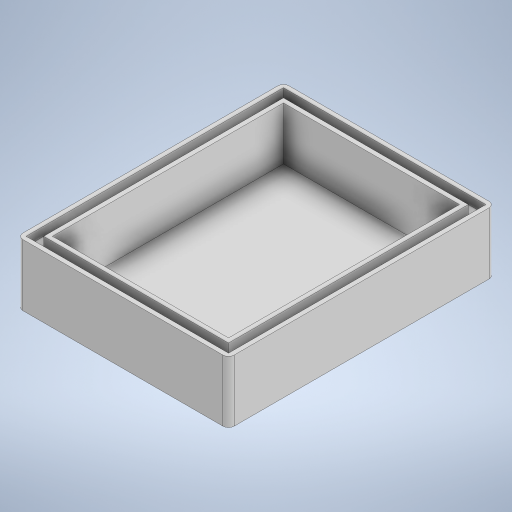
# Autodesk Inventor part: Light Sensor Box V1
Saved by Autodesk Inventor 2024.2 (Build 282272000, 272)
## iProperties
Created: 2024-07-12
Part Number: Light Sensor Box V1
Material: Generic
Document SubType Name: Modeling
Designer: balmo
Density: 1 g/cm^3
Appearance: Default
Author: balmo
## iProperties of the stored document Light Sensor Box V1_3DPrint.ipt
Created: 2024-07-12
Part Number: Light Sensor Box V1_3DPrint
Material: Generic
Document SubType Name: Modeling
Designer: balmo
Density: 1 g/cm^3
Appearance: Default
Author: balmo
Autodesk Inventor part; units mm, degrees
ref_plane "YZ Plane" through (0, 0, 0) normal (1, 0, 0) x (0, 1, 0)
ref_plane "XZ Plane" through (0, 0, 0) normal (0, 1, 0) x (-1, 0, 0)
ref_plane "XY Plane" through (0, 0, 0) normal (0, 0, 1) x (1, 0, 0)
sketch "Sketch1" plane through (0, 0, 0) normal (0, 1, 0) x (-1, 0, 0)
  line L0 (0, 0) -> (15.875, 0)
  line L1 (15.875, 0) -> (15.875, -20.828)
  line L2 (15.875, -20.828) -> (0, -20.828)
  line L3 (0, -20.828) -> (0, 0)
  line L4 (17.4625, 1.5875) -> (-1.5875, 1.5875)
  line L5 (-1.5875, 1.5875) -> (-1.5875, -22.4155)
  line L6 (-1.5875, -22.4155) -> (17.4625, -22.4155)
  line L7 (17.4625, -22.4155) -> (17.4625, 1.5875)
  dimension "d0" = 20.828
  dimension "d1" = 15.875
  dimension "d2" = 1.5875
  dimension "d3" = 1.5875
  dimension "d4" = 1.5875
  dimension "d5" = 1.5875
  constraints: 16 end point, 4 parallel, 2 horizontal, 2 perpendicular
  measures "d0" distance of L0.end L1.end
  measures "d1" distance of L1.end L2.end
  measures "d2" distance between parallel lines of L7 L1
  measures "d3" distance between parallel lines of L4 L0
  measures "d4" distance between parallel lines of L6 L2
  measures "d5" distance between parallel lines of L3 L5
extrude "Extrusion1" add sketch "Sketch1" along normal blind 0.7937 contours L0 L1 L2 L3
extrude "Extrusion2" add sketch "Sketch1" along normal blind 5.5563
sketch "Sketch2" plane through (0, 0.7937, 0) normal (0, 1, 0) x (1, 0, 0)
  line L0 (0, 0) -> (-15.875, 0) projected
  line L1 (0, 20.828) -> (-15.875, 20.828) projected
  line L2 (-15.875, 20.828) -> (-15.875, 0) projected
  line L3 (-15.875, 0) -> (0, 0) projected
  line L4 (0, 0) -> (0, 20.828) projected
  line L5 (-15.875, 0.7938) -> (0, 0.7937)
  line L6 (0, 0.7937) -> (0, 3.9688)
  line L7 (0, 3.9688) -> (-15.875, 3.9687)
  line L8 (-15.875, 3.9687) -> (-15.875, 0.7938)
  point P0 (0, 0.7937)
  dimension "d10" = 3.175
  dimension "d11" = 0.7937
  constraints: 8 end point, 2 parallel, 2 point on line, 1 horizontal, 1 perpendicular
  measures "d10" distance between parallel lines of L7 L5
  measures "d11" distance between parallel lines of L0 L5
extrude "Extrusion3" cut sketch "Sketch2" against normal blind 5.5563 contours L5 L2 L7 L4
sketch "Sketch3" plane through (0, 5.5563, 0) normal (0, 1, 0) x (1, 0, 0)
  line L0 (1.5875, -1.5875) -> (1.5875, 22.4155) projected
  line L1 (1.5875, 22.4155) -> (-17.4625, 22.4155) projected
  line L2 (-17.4625, 22.4155) -> (-17.4625, -1.5875) projected
  line L3 (-17.4625, -1.5875) -> (1.5875, -1.5875) projected
  line L4 (0, 0) -> (-15.875, 0) projected
  line L5 (-15.875, 0) -> (-15.875, 20.828) projected
  line L6 (-15.875, 20.828) -> (0, 20.828) projected
  line L7 (0, 20.828) -> (0, 0) projected
  line L8 (-17.0656, -1.1906) -> (1.1906, -1.1906)
  line L9 (1.1906, -1.1906) -> (1.1906, 22.0186)
  line L10 (1.1906, 22.0186) -> (-17.0656, 22.0186)
  line L11 (-17.0656, 22.0186) -> (-17.0656, -1.1906)
  line L12 (-16.2719, -0.3969) -> (0.3969, -0.3969)
  line L13 (0.3969, -0.3969) -> (0.3969, 21.2249)
  line L14 (0.3969, 21.2249) -> (-16.2719, 21.2249)
  line L15 (-16.2719, 21.2249) -> (-16.2719, -0.3969)
  dimension "d14" = 0.3969
  dimension "d15" = 0.3969
  dimension "d16" = 0.3969
  dimension "d17" = 0.3969
  dimension "d18" = 0.3969
  dimension "d19" = 0.3969
  dimension "d20" = 0.3969
  dimension "d21" = 0.3969
  constraints: 16 end point, 4 parallel, 2 horizontal, 2 perpendicular
  measures "d14" distance between parallel lines of L9 L0
  measures "d15" distance between parallel lines of L7 L13
  measures "d16" distance between parallel lines of L4 L12
  measures "d17" distance between parallel lines of L3 L8
  measures "d18" distance between parallel lines of L2 L11
  measures "d19" distance between parallel lines of L5 L15
  measures "d20" distance between parallel lines of L14 L6
  measures "d21" distance between parallel lines of L1 L10
extrude "Extrusion4" cut sketch "Sketch3" against normal blind 0.7937 contours L11 L10 L9 L8
fillet "Fillet1" radius 0.508 4 edges at (-17.4625, 2.7781, 1.5875) (-17.4625, 2.7781, -22.4155) (1.5875, 2.7781, -22.4155) (1.5875, 2.7781, 1.5875)
body "Solid1"
